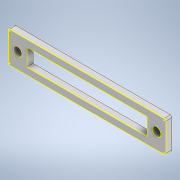
# Autodesk Inventor part: LED_Holder_BackBot
Saved by Autodesk Inventor 2021 (Build 250183000, 183)
## iProperties
Created: 2021-02-24
Part Number: LED_Holder_BackBot
Material: Generic
Document SubType Name: Modeling
Designer: Viktor
Density: 1 g/cm^3
Appearance: Default
Author: Viktor
Autodesk Inventor part; units mm, degrees
ref_plane "YZ Plane" through (0, 0, 0) normal (1, 0, 0) x (0, 1, 0)
ref_plane "XZ Plane" through (0, 0, 0) normal (0, 1, 0) x (-1, 0, 0)
ref_plane "XY Plane" through (0, 0, 0) normal (0, 0, 1) x (1, 0, 0)
sketch "Sketch1" plane through (0, 0, 0) normal (0, 0, 1) x (1, 0, 0)
  line L0 (-95, -10) -> (95, -10)
  line L1 (95, -10) -> (95, 10)
  line L2 (95, 10) -> (-95, 10)
  line L3 (-95, 10) -> (-95, -10)
  line L4 (-95, -10) -> (95, 10) construction
  line L5 (95, -10) -> (-95, 10) construction
  line L6 (-133, 0) -> (133, 0) construction
  line L7 (-83, -5.5) -> (-6, -5.5)
  line L8 (-6, -5.5) -> (-6, 5.5)
  line L9 (-6, 5.5) -> (-83, 5.5)
  line L10 (-83, 5.5) -> (-83, -5.5)
  line L11 (-83, -5.5) -> (-6, 5.5) construction
  line L12 (-6, -5.5) -> (-83, 5.5) construction
  line L13 (0, 14.2899) -> (0, -14.2899) construction
  line L14 (83, -5.5) -> (6, -5.5)
  line L15 (6, -5.5) -> (6, 5.5)
  line L16 (6, 5.5) -> (83, 5.5)
  line L17 (83, 5.5) -> (83, -5.5)
  line L18 (83, -5.5) -> (6, 5.5) construction
  line L19 (6, -5.5) -> (83, 5.5) construction
  circle A0 centre (-89, 0) radius 2.75
  circle A1 centre (0, 0) radius 2.75
  circle A2 centre (89, 0) radius 2.75
  line L20 (6, 5.5) -> (6, 10)
  line L21 (6, -5.5) -> (6, -10)
  point P0 (-44.5, 0)
  point P1 (44.5, 0)
  dimension "d0" = 190
  dimension "d1" = 20
  dimension "d2" = 11
  dimension "d3" = 12
  dimension "d4" = 6
  dimension "d5" = 5.5
  dimension "d6" = 6
  dimension "d7" = 5.5
  constraints: 40 end point, 6 midpoint, 6 symmetric about line, 5 point on line, 4 parallel, 3 centre point, 2 horizontal, 2 perpendicular, 1 coincident, 1 vertical, 1 other
  measures "d0" distance between parallel lines of L1 L3
  measures "d1" distance between parallel lines of L0 L2
  measures "d2" distance between parallel lines of L7 L9
  measures "d3" distance between parallel lines of L3 L10
  measures "d4" horizontal distance of point (0, 0) L8.end
  measures "d5" diameter of A0
  measures "d6" distance from line of L10 A0.centre
  measures "d7" diameter of A1
extrude "Extrusion1" add sketch "Sketch1" along normal blind 4 contours L3 L2 L20 L15 L21 L0
fillet "Fillet1" radius 1 4 edges at (-95, -10, 2) (-95, 10, 2) (6, -10, 2) (6, 10, 2)
sketch "Sketch2" plane through (0, 0, 4) normal (0, 0, 1) x (1, 0, 0)
  arc A0 (6, 9) -> (5, 10) centre (5, 9) ccw projected
  line L0 (5, 10) -> (-94, 10) projected
  arc A1 (-94, 10) -> (-95, 9) centre (-94, 9) ccw projected
  line L1 (-95, 9) -> (-95, -9) projected
  arc A2 (-95, -9) -> (-94, -10) centre (-94, -9) ccw projected
  line L2 (-94, -10) -> (5, -10) projected
  arc A3 (5, -10) -> (6, -9) centre (5, -9) ccw projected
  line L3 (6, -9) -> (6, 9) projected
  circle A4 centre (-89, 0) radius 2.75 projected
  circle A5 centre (0, 0) radius 2.75 projected
  line L4 (-83, -5.5) -> (-83, 5.5) projected
  line L5 (-83, 5.5) -> (-6, 5.5) projected
  line L6 (-6, 5.5) -> (-6, -5.5) projected
  line L7 (-6, -5.5) -> (-83, -5.5) projected
equation "\"d6\" = 0.5 * d3"
equation "\"d7\" = d5"
body "Solid1"
